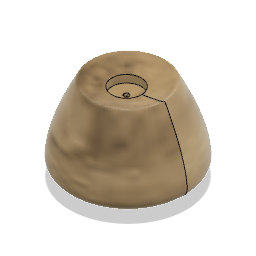
body_cam3v9 (Autodesk Fusion 360 design; units mm, degrees)
Autodesk Fusion 360 part; units mm, degrees
sketch "スケッチ1" plane through (0, 0, 0) normal (0, 0, 1) x (1, 0, 0)
  line L0 (0, 0) -> (0, 19.789099)
  spline S0 degree 5 poles (0, 19.789099) (0.06706, 19.790111) (0.202071, 19.791857) (0.407254, 19.793647) (0.686169, 19.794371) (1.043707, 19.792687) (1.410113, 19.788949) (1.78533, 19.784243) (2.16925, 19.780363) (2.561771, 19.779705) (2.962844, 19.785189) (3.372514, 19.800148) (3.790976, 19.828288) (4.21864, 19.872897) (4.656232, 19.935872) (5.104821, 20.01692) (5.566041, 20.112428) (6.041703, 20.21528) (6.531373, 20.317839) (7.030235, 20.414452) (7.526925, 20.504054) (8.001173, 20.592943) (8.422071, 20.696903) (8.760255, 20.828563) (8.999979, 20.984859) (9.150416, 21.135383) (9.259567, 21.207684) (9.389677, 21.119613) (9.581758, 20.825945) (9.850728, 20.323211) (10.193474, 19.63669) (10.592901, 18.812961) (11.023588, 17.910229) (11.456821, 16.989505) (11.865723, 16.105707) (12.23072, 15.298112) (12.543751, 14.583108) (12.805232, 13.960131) (13.021906, 13.416009) (13.204383, 12.929829) (13.364751, 12.477731) (13.514329, 12.037369) (13.660932, 11.593382) (13.807953, 11.139186) (13.955681, 10.674236) (14.102051, 10.202438) (14.243609, 9.730153) (14.376407, 9.264258) (14.496842, 8.810574) (14.602221, 8.373285) (14.691474, 7.954036) (14.76562, 7.551353) (14.828807, 7.159445) (14.887293, 6.769138) (14.946257, 6.371037) (15.007287, 5.958012) (15.065354, 5.528144) (15.106685, 5.086956) (15.113356, 4.64443) (15.067523, 4.212364) (14.955348, 3.801817) (14.772121, 3.419997) (14.52283, 3.069378) (14.217679, 2.74933) (13.868871, 2.457098) (13.487031, 2.189007) (13.07739, 1.94166) (12.640581, 1.712072) (12.174074, 1.497623) (11.673424, 1.296081) (11.133504, 1.105595) (10.549959, 0.924706) (9.919662, 0.75232) (9.240382, 0.58765) (8.510689, 0.430165) (7.729753, 0.279544) (7.063708, 0.164407) (6.540902, 0.081042) (6.182024, 0.026793) (6, 0) knots 0 0 0 0 0 0 0.01333333 0.02666667 0.04 0.05333333 0.06666667 0.08 0.09333333 0.10666667 0.12 0.13333333 0.14666667 0.16 0.17333333 0.18666667 0.2 0.21333333 0.22666667 0.24 0.25333333 0.26666667 0.28 0.29333333 0.30666667 0.32 0.33333333 0.34666667 0.36 0.37333333 0.38666667 0.4 0.41333333 0.42666667 0.44 0.45333333 0.46666667 0.48 0.49333333 0.50666667 0.52 0.53333333 0.54666667 0.56 0.57333333 0.58666667 0.6 0.61333333 0.62666667 0.64 0.65333333 0.66666667 0.68 0.69333333 0.70666667 0.72 0.73333333 0.74666667 0.76 0.77333333 0.78666667 0.8 0.81333333 0.82666667 0.84 0.85333333 0.86666667 0.88 0.89333333 0.90666667 0.92 0.93333333 0.94666667 0.96 0.97333333 0.98666667 1 1 1 1 1 1
  line L1 (6, 0) -> (0, 0)
  point P0 (1.377048, 19.789099)
  point P1 (3.020853, 19.789099)
  point P2 (5, 20)
  point P3 (7.5, 20.5)
  point P4 (9, 21)
  point P5 (9.306638, 21.154855)
  point P6 (11.791503, 16.262776)
  point P7 (13.44574, 12.237325)
  point P8 (14.193466, 9.89455)
  point P9 (14.727556, 7.750969)
  point P10 (15, 6)
  point P11 (15, 4)
  point P12 (13.814209, 2.42788)
  point P13 (11.430505, 1.21354)
  constraint coincident L0.start L1.end
  constraint vertical L0
  constraint perpendicular L0 L1
revolve "回転1" add sketch "スケッチ1" angle 360 about axis through (0, 0, 0) along (0, 1, 0) contours L0 S0 L1 picked at (7.404057, 10.826669) makes body 1
sketch "スケッチ2" plane through (0, 0, 0) normal (0, 0, 1) x (1, 0, 0)
sketch "スケッチ3" plane through (0, 0, 0) normal (1, 0, 0) x (0, 0, -1)
sketch "スケッチ5" plane through (0, 0, 0) normal (0, 1, 0) x (1, 0, 0)
move_body "移動1" bodies 1 to x (1, 0, 0) y (0, 1, 0) z (0, 0, 1) at (0, -19.789099, 0)
move_body "移動3" bodies 1 to x (1, 0, 0) y (0, 1, 0) z (0, 0, 1) at (0, 19.789099, 0)
hole "穴4" at (-0.158505, 19.792266, 0.220718) direction (-0.00484, -0.999966, 0.006739) diameter 1.3 depth 7 tip angle 180 bodies 1
sketch "スケッチ7" plane through (0, 0, 0) normal (0, 0, 1) x (1, 0, 0)
sketch "スケッチ8" plane through (0, 0, 0) normal (0, 0, 1) x (1, 0, 0)
  spline S0 degree 5 poles (-39.809152, 19.668003) (-39.763341, 19.664704) (-39.661615, 19.659168) (-39.478718, 19.654049) (-39.174215, 19.653597) (-38.694394, 19.664113) (-38.121154, 19.687052) (-37.466311, 19.725118) (-36.745986, 19.781806) (-35.978748, 19.860808) (-35.183755, 19.965409) (-34.378995, 20.097934) (-33.579241, 20.259032) (-32.79585, 20.448054) (-32.037093, 20.663736) (-31.308284, 20.904782) (-30.612005, 21.170481) (-29.948265, 21.461326) (-29.314728, 21.779587) (-28.707909, 22.128675) (-28.124308, 22.51258) (-27.561604, 22.935277) (-27.019747, 23.400137) (-26.5023, 23.909361) (-26.01526, 24.463203) (-25.565607, 25.059223) (-25.159882, 25.691405) (-24.802886, 26.349605) (-24.496001, 27.018171) (-24.23702, 27.6777) (-24.02129, 28.309354) (-23.842482, 28.898703) (-23.693509, 29.439227) (-23.56739, 29.937293) (-23.458092, 30.410795) (-23.361425, 30.882718) (-23.275761, 31.376473) (-23.203207, 31.909813) (-23.148316, 32.493322) (-23.115724, 33.130287) (-23.108367, 33.816335) (-23.124927, 34.538654) (-23.15936, 35.27706) (-23.204582, 36.009049) (-23.255365, 36.714095) (-23.311378, 37.378061) (-23.380574, 37.998023) (-23.48127, 38.585606) (-23.634892, 39.159508) (-23.859179, 39.738727) (-24.162181, 40.336296) (-24.533521, 40.950914) (-24.947092, 41.567578) (-25.372114, 42.164938) (-25.782265, 42.720943) (-26.164482, 43.218609) (-26.530664, 43.653144) (-26.918199, 44.03342) (-27.374661, 44.375336) (-27.946477, 44.697215) (-28.665851, 45.014327) (-29.538825, 45.333945) (-30.550574, 45.656859) (-31.670314, 45.978769) (-32.856353, 46.291718) (-34.061006, 46.58549) (-35.235679, 46.84905) (-36.335601, 47.071892) (-37.325373, 47.245605) (-38.182029, 47.364767) (-38.891753, 47.426127) (-39.336611, 47.427726) (-39.600139, 47.401993) (-39.744673, 47.372873) (-39.809152, 47.355321) knots 0 0 0 0 0 0 0.01428571 0.02857143 0.04285714 0.05714286 0.07142857 0.08571429 0.1 0.11428571 0.12857143 0.14285714 0.15714286 0.17142857 0.18571429 0.2 0.21428571 0.22857143 0.24285714 0.25714286 0.27142857 0.28571429 0.3 0.31428571 0.32857143 0.34285714 0.35714286 0.37142857 0.38571429 0.4 0.41428571 0.42857143 0.44285714 0.45714286 0.47142857 0.48571429 0.5 0.51428571 0.52857143 0.54285714 0.55714286 0.57142857 0.58571429 0.6 0.61428571 0.62857143 0.64285714 0.65714286 0.67142857 0.68571429 0.7 0.71428571 0.72857143 0.74285714 0.75714286 0.77142857 0.78571429 0.8 0.81428571 0.82857143 0.84285714 0.85714286 0.87142857 0.88571429 0.9 0.91428571 0.92857143 0.94285714 0.95714286 0.97142857 0.98571429 1 1 1 1 1 1
  line L0 (-39.809152, 47.355321) -> (-39.809152, 19.668003)
  point P0 (-38.647348, 19.668003)
  point P1 (-35.000001, 20)
  point P2 (-30.656979, 21.161751)
  point P3 (-27.5, 23)
  point P4 (-23.780994, 29.12841)
  point P5 (-23.338836, 31.026417)
  point P6 (-23.114176, 33.59396)
  point P7 (-23.306742, 37.284805)
  point P8 (-24, 40.000001)
  point P9 (-26, 43.000001)
  point P10 (-27.96348, 44.686182)
  point P11 (-36.000001, 47.000001)
  constraint vertical L0
extrude "押し出し2" cut 1 faces at (-0.390854, 19.791735, -0.024937) along direction (-0.0048398, -0.99996558, 0.00673939) blind 0.555 and the other way blind 0.762 on bodies 1 bodies 1
copy_body "ボディ -> コンポーネント1" bodies 1 removing the originals makes body 2 in component "Component"
move_face "面を移動1" to x (1, 0, 0) y (0, 1, 0) z (0, 0, 1) at (-0.450926, 4.80988, 0) 1 faces at (12.393621, 14.714017, -1.502626) on bodies 2 in component "Component"
move_face "面を移動2" to x (1, 0, 0) y (0, 1, 0) z (0, 0, 1) at (0, 0, 0) 1 faces at (12.393621, 14.714017, -1.502626) on bodies 2 in component "Component"
move_face "面を移動3" to x (1, 0, 0) y (0, 1, 0) z (0, 0, 1) at (0.526081, 4.80988, 0) 1 faces at (12.393621, 14.714017, -1.502626) on bodies 2 in component "Component"
move_body "移動1'" bodies 2 to x (1, 0, 0) y (0, 1, 0) z (0, 0, 1) at (0, 4.133491, 0) in component "Component"
move_body "移動2" bodies 2 to x (1, 0, 0) y (0, 1, 0) z (0, 0, 1) at (0, 0, 4) in component "Component"
move_body "移動3'" bodies 2 to x (1, 0, 0) y (0, 1, 0) z (0, 0, 1) at (-0.375772, -1.427933, 0) in component "Component"
scale "尺度1" factor 2 about (0, 0, 0) bodies 2 in component "Component"
move_body "移動4" bodies 2 to x (1, 0, 0) y (0, 1, 0) z (0, 0, 1) at (0, -2.743503, 0) in component "Component"
scale "尺度2" factor 0.8 about (11.248456, 2.667613, 8) bodies 2 in component "Component"
move_body "移動5" bodies 2 to x (1, 0, 0) y (0, 1, 0) z (0, 0, 1) at (-1.969616, 0, -0.347296) in component "Component"
sketch "スケッチ9" plane through (0, 0, 0) normal (0, 1, 0) x (1, 0, 0)
  circle A0 through (5.915577, -10.167183, 32.045962) (-3.084423, -4.971031, 32.045962) (-3.084423, -15.363336, 32.045962)
extrude "押し出し1" cut sketch "スケッチ9" against normal blind 3.3 contours A0 in plane through (0, 32.046, 0) normal (0, 1, 0) picked at (-3.815105, 32.046, 10.29688) sketch seen with x (1, 0, 0) y (0, 1, 0) z (0, 0, 1) at (-0.450255, 2.61298, -2.162725) bodies 2 in component "Component"
hole "穴2" at (-0.582088, 31.358942, 8.036065) direction (0, -1, 0) diameter 2.1 depth 7 tip angle 118 bodies 2 in component "Component"
component "Component" placed x (1, 0, 0) y (0, 1, 0) z (0, 0, 1) at (0.450255, -2.61298, 2.162725)
